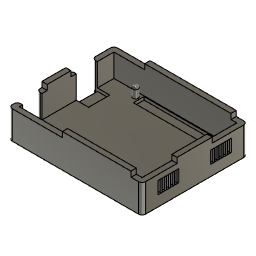
arduino-box-v3 (Autodesk Fusion 360 design; units mm, degrees)
Autodesk Fusion 360 part; units mm, degrees
note: some values were not read from the file. Set by a fixed rule: which sketch regions a step uses.
sketch "Base" plane through (0, 0, 0) normal (0, 0, 1) x (1, 0, 0)
  line L0 (0, 0) -> (75.8, 0)
  line L1 (75.8, 0) -> (75.8, 59.8)
  line L2 (75.8, 59.8) -> (0, 59.8)
  line L3 (0, 59.8) -> (0, 0)
  line L4 (3, 3) -> (72.8, 3)
  line L5 (72.8, 3) -> (72.8, 56.8)
  line L6 (72.8, 56.8) -> (3, 56.8)
  line L7 (3, 56.8) -> (3, 3)
  line L8 (3, 56.8) -> (3, 59.8) construction
  line L9 (3, 56.8) -> (0, 56.8) construction
  line L10 (72.8, 3) -> (72.8, 0) construction
  line L11 (75.8, 3) -> (72.8, 3) construction
  line L12 (3.4, 3.4) -> (72.4, 3.4)
  line L13 (72.4, 3.4) -> (72.4, 56.4)
  line L14 (72.4, 56.4) -> (3.4, 56.4)
  line L15 (3.4, 56.4) -> (3.4, 3.4)
  line L16 (3.4, 56.4) -> (3, 56.4) construction
  line L17 (3.4, 56.4) -> (3.4, 56.8) construction
  line L18 (72.4, 3.4) -> (72.4, 3) construction
  line L19 (72.4, 3.4) -> (72.8, 3.4) construction
  line L20 (3, 13.4) -> (13, 13.4)
  line L21 (13, 13.4) -> (13, 3.4)
  line L22 (0, 15.9) -> (3, 15.9)
  line L23 (0, 4.9) -> (3, 4.9)
  line L24 (0, 47.4) -> (3, 47.4)
  line L25 (0, 35.4) -> (3, 35.4)
  line L26 (3, 47.4) -> (10, 47.4)
  line L27 (10, 47.4) -> (10, 35.4)
  line L28 (10, 35.4) -> (3, 35.4)
  line L29 (20.5, 56.4) -> (20.5, 50.4)
  line L30 (20.5, 50.4) -> (69.5, 50.4)
  line L31 (69.5, 50.4) -> (69.5, 56.4)
  line L32 (30.5, 3.4) -> (30.5, 9.4)
  line L33 (30.5, 9.4) -> (69.5, 9.4)
  line L34 (69.5, 9.4) -> (69.5, 3.4)
  line L35 (72.4, 35.4) -> (66.4, 35.4)
  line L36 (66.4, 35.4) -> (66.4, 26.4)
  line L37 (66.4, 26.4) -> (72.4, 26.4)
  circle A0 centre (18.2, 53.86) radius 1.5
  circle A1 centre (70, 38.4) radius 1.5
  circle A2 centre (70, 10.4) radius 1.5
  line L38 (3.4, 3.4) -> (3, 3.4)
  dimension "d9" = 3
  dimension "d10" = 0.4
  dimension "d11" = 53
  dimension "d12" = 69
  dimension "charging_hole_length" = 10
  dimension "charging_space" = 11
  dimension "charging_y_coord" = 4.9
  dimension "usb_space" = 12
  dimension "usb_y_coord" = 35.4
  dimension "usb_hole_length" = 7
  dimension "d19" = 6
  dimension "pin_row_1_length" = 49
  dimension "pin_row_1_x_coord" = 20.5
  dimension "d22" = 6
  dimension "pin_row_2_length" = 39
  dimension "pin_row_2_x_coord" = 30.5
  dimension "centered_pins_length" = 9
  dimension "d26" = 6
  dimension "centered_pins_y_coord" = 26.4
  dimension "d28" = 3
  dimension "circle_1_x_coord" = 18.2
  dimension "circle_1_space_to_top" = 2.54
  dimension "circle_2_y_coord" = 38.4
  dimension "circle_3_y_coord" = 10.4
  dimension "circle_2_x_coord" = 70
  dimension "circle_3_x_coord" = 70
  constraint horizontal L0
  constraint vertical L1
  constraint horizontal L2
  constraint vertical L3
  constraint coincident L0.start L3.end
  constraint horizontal L4
  constraint vertical L5
  constraint horizontal L6
  constraint vertical L7
  constraint coincident L2 L8.end
  constraint perpendicular L6 L8
  constraint coincident L3 L9.end
  constraint perpendicular L3 L9
  constraint coincident L0 L10.end
  constraint perpendicular L0 L10
  constraint coincident L1 L11.start
  constraint perpendicular L5 L11
  constraint equal L8 L9
  constraint equal L8 L11
  constraint equal L8 L10
  constraint horizontal L12
  constraint vertical L13
  constraint horizontal L14
  constraint vertical L15
  constraint coincident L7 L16.end
  constraint perpendicular L7 L16
  constraint coincident L6 L17.end
  constraint perpendicular L6 L17
  constraint coincident L4 L18.end
  constraint perpendicular L4 L18
  constraint coincident L5 L19.end
  constraint perpendicular L5 L19
  constraint equal L16 L17
  constraint equal L17 L19
  constraint equal L17 L18
  constraint coincident L7 L20.start
  constraint perpendicular L15 L20
  constraint coincident L12 L21.end
  constraint perpendicular L12 L21
  constraint equal L20 L21
  constraint coincident L3 L22.start
  constraint coincident L7 L22.end
  constraint perpendicular L7 L22
  constraint coincident L3 L23.start
  constraint coincident L7 L23.end
  constraint perpendicular L7 L23
  constraint coincident L3 L24.start
  constraint coincident L7 L24.end
  constraint perpendicular L7 L24
  constraint coincident L3 L25.start
  constraint coincident L7 L25.end
  constraint perpendicular L7 L25
  constraint perpendicular L15 L26
  constraint perpendicular L26 L27
  constraint perpendicular L27 L28
  constraint coincident L14 L29.start
  constraint perpendicular L14 L29
  constraint perpendicular L29 L30
  constraint coincident L14 L31.end
  constraint perpendicular L30 L31
  constraint coincident L12 L32.start
  constraint perpendicular L12 L32
  constraint perpendicular L3 L33
  constraint coincident L12 L34.end
  constraint perpendicular L33 L34
  constraint coincident L13 L35.start
  constraint perpendicular L13 L35
  constraint perpendicular L35 L36
  constraint coincident L13 L37.end
  constraint perpendicular L13 L37
  constraint equal A0 A2
  constraint equal A0 A1
  constraint coincident L7 L38.end
  constraint perpendicular L7 L38
  measures "d9" distance of L6.end L8.end
  measures "d10" distance of L14.end L17.end
  measures "d11" distance of L12.start L14.end
  measures "d12" distance of L13.end L14.end
  measures "charging_hole_length" distance of L20.start L20.end
  measures "charging_space" distance of L22 L23
  measures "charging_y_coord" distance of L0 L23
  measures "usb_space" distance of L24 L25
  measures "usb_y_coord" distance of L0 L25
  measures "usb_hole_length" distance of L24.end L26.end
  measures "d19" distance of L30.end L31.end
  measures "pin_row_1_length" distance of L29.end L30.end
  measures "pin_row_1_x_coord" distance of L3 L29
  measures "d22" distance of L33.end L34.end
  measures "pin_row_2_length" distance of L32.end L33.end
  measures "pin_row_2_x_coord" distance of L3 L32
  measures "centered_pins_length" distance of L35.end L36.end
  measures "d26" distance of L35.start L35.end
  measures "centered_pins_y_coord" distance of L0 L37
  measures "d28" diameter of A0
  measures "circle_1_x_coord" distance of L3 A0.centre
  measures "circle_1_space_to_top" distance of L14 A0.centre
  measures "circle_2_y_coord" distance of L0 A1.centre
  measures "circle_3_y_coord" distance of L0 A2.centre
  measures "circle_2_x_coord" distance of L3 A1.centre
  measures "circle_3_x_coord" distance of L3 A2.centre
extrude "Extrude1" add sketch "Base" along normal blind 3 contours L7 L15 L20 L28 | L4 L5 L6 L7 L12 L13 L14 L15 L26 L38 | L12 L13 L14 L15 L20 L21 L26 L27 L28 L29 L30 L31 L32 L33 L34 L35 L36 L37 A2
extrude "Extrude2" add sketch "Base" along normal blind 16 contours L0 L1 L2 L3 L4 L5 L6 L7 L23 L24 | L3 L7 L22 L25
extrude "Extrude3" add sketch "Base" along normal blind 1.3 contours L7 L15 L20 L38 | L7 L15 L26 L28 | L12 L15 L20 L21 | L15 L26 L27 L28 | L12 L32 L33 L34 A2 | L14 L29 L30 L31 | L13 L35 L36 L37
extrude "Extrude4" add sketch "Base" along normal blind 9 contours L33 L34 A2 | L33 L34 A2 | A0 | A1
sketch "Ventilation" plane through (75.8, 0, 0) normal (1, 0, 0) x (0, 1, 0)
  line L0 (0, 0) -> (59.8, 0)
  line L1 (59.8, 0) -> (59.8, 16)
  line L2 (59.8, 16) -> (0, 16)
  line L3 (0, 16) -> (0, 0)
  line L4 (0, 3) -> (59.8, 3) construction
  line L5 (0, 0) -> (59.8, 0)
  line L6 (29.9, 16) -> (29.9, 3) construction
  line L7 (29.9, 9.5) -> (0, 9.5) construction
  line L8 (15.55, 13) -> (14.35, 13)
  line L9 (14.35, 13) -> (14.35, 6)
  line L10 (14.35, 6) -> (15.55, 6)
  line L11 (15.55, 6) -> (15.55, 13)
  line L12 (15.55, 13) -> (14.35, 6) construction
  line L13 (14.35, 13) -> (15.55, 6) construction
  line L14 (15.55, 13) -> (16.75, 13) construction
  line L15 (16.75, 13) -> (17.95, 13)
  line L16 (17.95, 13) -> (17.95, 6)
  line L17 (17.95, 6) -> (16.75, 6)
  line L18 (16.75, 6) -> (16.75, 13)
  line L19 (17.95, 13) -> (19.15, 13) construction
  line L20 (19.15, 13) -> (20.35, 13)
  line L21 (20.35, 13) -> (20.35, 6)
  line L22 (20.35, 6) -> (19.15, 6)
  line L23 (19.15, 6) -> (19.15, 13)
  line L24 (14.35, 13) -> (13.15, 13) construction
  line L25 (13.15, 13) -> (11.95, 13)
  line L26 (11.95, 13) -> (11.95, 6)
  line L27 (11.95, 6) -> (13.15, 6)
  line L28 (13.15, 6) -> (13.15, 13)
  line L29 (11.95, 13) -> (10.75, 13) construction
  line L30 (10.75, 13) -> (9.55, 13)
  line L31 (9.55, 13) -> (9.55, 6)
  line L32 (9.55, 6) -> (10.75, 6)
  line L33 (10.75, 6) -> (10.75, 13)
  line L34 (40.65, 13) -> (39.45, 13)
  line L35 (40.65, 6) -> (40.65, 13)
  line L36 (39.45, 13) -> (39.45, 6)
  line L37 (39.45, 6) -> (40.65, 6)
  line L38 (41.85, 13) -> (41.85, 6)
  line L39 (41.85, 6) -> (43.05, 6)
  line L40 (43.05, 6) -> (43.05, 13)
  line L41 (43.05, 13) -> (41.85, 13)
  line L42 (44.25, 6) -> (44.25, 13)
  line L43 (45.45, 13) -> (45.45, 6)
  line L44 (45.45, 6) -> (44.25, 6)
  line L45 (44.25, 13) -> (45.45, 13)
  line L46 (46.65, 6) -> (46.65, 13)
  line L47 (47.85, 13) -> (47.85, 6)
  line L48 (46.65, 13) -> (47.85, 13)
  line L49 (49.05, 13) -> (50.25, 13)
  line L50 (49.05, 6) -> (49.05, 13)
  line L51 (50.25, 13) -> (50.25, 6)
  line L52 (50.25, 6) -> (49.05, 6)
  line L53 (47.85, 6) -> (46.65, 6)
  point P0 (14.95, 9.5)
  dimension "d43" = 3
  dimension "ventilation_height" = 7
  dimension "ventilation_width" = 1.2
  constraint coincident L3 L4.start
  constraint coincident L1 L4.end
  constraint perpendicular L1 L4
  constraint midpoint L2 L6.start
  constraint midpoint L4 L6.end
  constraint midpoint L6 L7.start
  constraint coincident L3 L7.end
  constraint perpendicular L6 L7
  constraint horizontal L8
  constraint perpendicular L8 L9
  constraint parallel L8 L10
  constraint parallel L9 L11
  constraint coincident L12 P0
  constraint coincident L13 P0
  constraint midpoint L7 P0
  constraint perpendicular L11 L14
  constraint horizontal L15
  constraint vertical L16
  constraint horizontal L17
  constraint vertical L18
  constraint perpendicular L16 L19
  constraint horizontal L20
  constraint vertical L21
  constraint horizontal L22
  constraint vertical L23
  constraint perpendicular L9 L24
  constraint horizontal L25
  constraint vertical L26
  constraint horizontal L27
  constraint vertical L28
  constraint perpendicular L26 L29
  constraint horizontal L30
  constraint vertical L31
  constraint horizontal L32
  constraint vertical L33
  constraint equal L8 L30
  constraint equal L8 L29
  constraint equal L8 L25
  constraint equal L8 L24
  constraint coincident L14.end L15.start
  constraint equal L8 L14
  constraint equal L8 L15
  constraint equal L8 L19
  constraint equal L8 L20
  constraint equal L9 L28
  constraint equal L9 L33
  constraint equal L11 L18
  constraint equal L11 L23
  constraint symmetric L6 L8.start L42.end
  constraint symmetric L6 L8.end L43.start
  constraint symmetric L6 L9.end L43.end
  constraint symmetric L6 L10.end L42.start
  constraint symmetric L6 L14.end L40.end
  constraint symmetric L6 L15.end L38.start
  constraint symmetric L6 L16.end L38.end
  constraint symmetric L6 L17.end L39.end
  constraint symmetric L6 L19.end L34.start
  constraint symmetric L6 L20.end L34.end
  constraint symmetric L6 L21.end L36.end
  constraint symmetric L6 L22.end L35.start
  constraint symmetric L6 L24.end L46.end
  constraint symmetric L6 L25.end L47.start
  constraint symmetric L6 L26.end L47.end
  constraint symmetric L6 L27.end L46.start
  constraint symmetric L6 L29.end L49.start
  constraint symmetric L6 L30.end L49.end
  constraint symmetric L6 L31.end L51.end
  constraint symmetric L6 L32.end L50.start
  measures "d43" distance of L4 L5
  measures "ventilation_height" distance of L8.end L9.end
  measures "ventilation_width" distance of L8.start L8.end
extrude "Extrude5" cut sketch "Ventilation" against normal blind 3 contours L8 L9 L10 L11 | L15 L16 L17 L18 | L20 L21 L22 L23 | L25 L26 L27 L28 | L30 L31 L32 L33 | L34 L35 L36 L37 | L38 L39 L40 L41 | L42 L43 L44 L45 | L46 L47 L48 L53 | L49 L50 L51 L52
fillet "Fillet1" radius 0.5 40 edges at (75.8, 20.35, 9.5) (75.8, 19.15, 9.5) (75.8, 17.95, 9.5) (72.8, 20.35, 9.5) (75.8, 16.75, 9.5) (72.8, 19.15, 9.5) (75.8, 15.55, 9.5) (72.8, 17.95, 9.5) (72.8, 16.75, 9.5) (75.8, 14.35, 9.5) (75.8, 13.15, 9.5) (72.8, 15.55, 9.5) (75.8, 11.95, 9.5) (72.8, 14.35, 9.5) (75.8, 10.75, 9.5) (72.8, 13.15, 9.5) (75.8, 9.55, 9.5) (72.8, 11.95, 9.5) (72.8, 10.75, 9.5) (72.8, 9.55, 9.5) (75.8, 50.25, 9.5) (75.8, 49.05, 9.5) (72.8, 50.25, 9.5) (75.8, 47.85, 9.5) (72.8, 49.05, 9.5) (75.8, 46.65, 9.5) (72.8, 47.85, 9.5) (75.8, 45.45, 9.5) (72.8, 46.65, 9.5) (75.8, 44.25, 9.5) (72.8, 45.45, 9.5) (75.8, 43.05, 9.5) (72.8, 44.25, 9.5) (75.8, 41.85, 9.5) (72.8, 43.05, 9.5) (75.8, 40.65, 9.5) (72.8, 41.85, 9.5) (75.8, 39.45, 9.5) (72.8, 40.65, 9.5) (72.8, 39.45, 9.5)
sketch "Teeth" plane through (0, 0, 16) normal (0, 0, 1) x (-1, 0, 0)
  line L0 (0, -4.9) -> (0, 0)
  line L1 (0, 0) -> (-75.8, 0)
  line L2 (-75.8, 0) -> (-75.8, -59.8)
  line L3 (-75.8, -59.8) -> (0, -59.8)
  line L4 (0, -59.8) -> (0, -47.4)
  line L5 (0, -47.4) -> (-3, -47.4)
  line L6 (-3, -47.4) -> (-3, -56.8)
  line L7 (-3, -56.8) -> (-72.8, -56.8)
  line L8 (-72.8, -56.8) -> (-72.8, -3)
  line L9 (-72.8, -3) -> (-3, -3)
  line L10 (-3, -3) -> (-3, -4.9)
  line L11 (-3, -4.9) -> (0, -4.9)
  line L12 (-20.5, -59.8) -> (-20.5, -56.8)
  line L13 (-69.5, -59.8) -> (-69.5, -56.8)
  line L14 (0, -59.8) -> (0, 0)
  line L15 (-20.5, -59.8) -> (-69.5, -59.8)
  line L16 (-20.5, -56.8) -> (-69.5, -56.8)
  line L17 (-72.8, -39.9) -> (-75.8, -39.9)
  line L18 (-75.8, -39.9) -> (-75.8, -19.9)
  line L19 (-75.8, -19.9) -> (-72.8, -19.9)
  line L20 (-72.8, -19.9) -> (-72.8, -39.9)
  line L21 (-75.8, 0) -> (-75.8, -59.8)
  line L22 (0, -32.4) -> (-3, -32.4)
  line L23 (-3, -32.4) -> (-3, -18.9)
  line L24 (-3, -18.9) -> (0, -18.9)
  line L25 (0, -32.4) -> (0, -18.9)
  line L26 (-30.5, 0) -> (-30.5, -3)
  line L27 (-30.5, -3) -> (-69.5, -3)
  line L28 (-69.5, -3) -> (-69.5, 0)
  line L29 (-69.5, 0) -> (-30.5, 0)
  point P0 (0, -35.4)
  point P1 (0, -15.9)
  dimension "d52" = 49
  dimension "d53" = 20.5
  dimension "back_tooth_length" = 20
  dimension "d55" = 3
  dimension "front_tooth_padding" = 3
  dimension "d57" = 3
  dimension "d58" = 39
  dimension "d59" = 30.5
  constraint coincident L3 L12.start
  constraint coincident L7 L12.end
  constraint perpendicular L7 L12
  constraint coincident L3 L13.start
  constraint coincident L7 L13.end
  constraint perpendicular L7 L13
  constraint horizontal L17
  constraint vertical L18
  constraint horizontal L19
  constraint vertical L20
  constraint coincident L2 L18.end
  constraint coincident L8 L17.start
  constraint midpoint L18 L21
  constraint coincident L14 L22.start
  constraint perpendicular L14 L22
  constraint coincident L14 L24.end
  constraint perpendicular L14 L24
  constraint perpendicular L23 L24
  constraint coincident L1 L26.start
  constraint coincident L9 L26.end
  constraint perpendicular L9 L26
  constraint coincident L9 L27.end
  constraint perpendicular L26 L27
  constraint coincident L1 L28.end
  constraint perpendicular L1 L28
  measures "d52" distance of L12 L13
  measures "d53" distance of L12 L14
  measures "back_tooth_length" distance of L17 L19
  measures "d55" distance of L22.start L22.end
  measures "front_tooth_padding" distance of L22 P0
  measures "d57" distance of L24 P1
  measures "d58" distance of L26 L28
  measures "d59" distance of L14 L26
extrude "Extrude6" add sketch "Teeth" along normal blind 3 contours L14 L22 L23 L24 L25 | L1 L9 L26 L27 L28 L29 | L2 L8 L17 L18 L19 L20 L21 | L3 L7 L12 L13 L15 L16
sketch "Plexi" plane through (0, 0, 16) normal (0, 0, 1) x (-1, 0, 0)
  line L0 (-20.5, -56.8) -> (-20.5, -59.8)
  line L1 (-20.5, -59.8) -> (0, -59.8)
  line L2 (0, -59.8) -> (0, -47.4)
  line L3 (0, -47.4) -> (-3, -47.4)
  line L4 (-3, -47.4) -> (-3, -56.8)
  line L5 (-3, -56.8) -> (-20.5, -56.8)
  line L6 (0, -32.4) -> (0, -59.8)
  line L7 (0, -59.8) -> (-20.5, -59.8)
  line L8 (-20.5, -59.8) -> (-20.5, -50.4)
  line L9 (-20.5, -50.4) -> (-69.5, -50.4)
  line L10 (-69.5, -50.4) -> (-69.5, -59.8)
  line L11 (-69.5, -59.8) -> (-75.8, -59.8)
  line L12 (-75.8, -59.8) -> (-75.8, -39.9)
  line L13 (-75.8, -39.9) -> (-72.8, -39.9)
  line L14 (-72.8, -39.9) -> (-72.8, -35.4)
  line L15 (-72.8, -35.4) -> (-66.4, -35.4)
  line L16 (-66.4, -35.4) -> (-66.4, -26.4)
  line L17 (-66.4, -26.4) -> (-72.8, -26.4)
  line L18 (-72.8, -26.4) -> (-72.8, -19.9)
  line L19 (-72.8, -19.9) -> (-75.8, -19.9)
  line L20 (-75.8, -19.9) -> (-75.8, 0)
  line L21 (-75.8, 0) -> (-69.5, 0)
  line L22 (-69.5, 0) -> (-69.5, -9.4)
  line L23 (-69.5, -9.4) -> (-30.5, -9.4)
  line L24 (-30.5, -9.4) -> (-30.5, 0)
  line L25 (-30.5, 0) -> (0, 0)
  line L26 (0, 0) -> (0, -18.9)
  line L27 (0, -18.9) -> (-3, -18.9)
  line L28 (-3, -18.9) -> (-3, -32.4)
  line L29 (-3, -32.4) -> (0, -32.4)
  point P0 (-75.8, -59.8)
  point P1 (-69.5, -59.8)
  point P2 (-69.5, -50.4)
  point P3 (-3, -32.4)
  point P4 (-3, -18.9)
  point P5 (-30.5, -9.4)
  point P6 (-69.5, 0)
  point P7 (-75.8, 0)
  point P8 (-72.8, -19.9)
  point P9 (-66.4, -26.4)
  point P10 (-72.8, -39.9)
  point P11 (-66.4, -35.4)
  constraint coincident L1.end L2.start
  constraint coincident L0.end L1.start
  constraint perpendicular L7 L8
  constraint perpendicular L8 L9
  constraint perpendicular L9 L10
  constraint perpendicular L10 L11
  constraint perpendicular L11 L12
  constraint perpendicular L10 L13
  constraint perpendicular L13 L14
  constraint perpendicular L14 L15
  constraint perpendicular L15 L16
  constraint perpendicular L16 L17
  constraint perpendicular L17 L18
  constraint perpendicular L18 L19
  constraint perpendicular L19 L20
  constraint perpendicular L20 L21
  constraint perpendicular L19 L22
  constraint perpendicular L20 L23
  constraint perpendicular L23 L24
  constraint coincident L25.end L26.start
  constraint perpendicular L24 L25
  constraint perpendicular L25 L26
  constraint perpendicular L26 L27
  constraint perpendicular L27 L28
  constraint perpendicular L28 L29
  constraint vertical L6
  constraint coincident L6.start L29.end
  constraint coincident P0 L11.end
  constraint coincident P1 L10.end
  constraint coincident P2 L9.end
  constraint coincident P3 L28.end
  constraint coincident P4 L27.end
  constraint coincident P5 L23.end
  constraint coincident P6 L21.end
  constraint coincident P7 L20.end
  constraint coincident P8 L18.end
  constraint coincident P9 L16.end
  constraint coincident P10 L13.end
  constraint coincident P11 L15.end
fillet "Fillet2" radius 2 8 edges at (0, 0, 8) (0, 4.9, 8) (0, 15.9, 8) (0, 35.4, 8) (0, 47.4, 8) (0, 59.8, 8) (75.8, 59.8, 8) (75.8, 0, 8)
fillet "Fillet3" radius 1.5 3 edges at (68.6015, 37.8576, 9) (68.6015, 9.8576, 9) (16.8015, 53.3176, 9)
equation "arduino_length = 69 mm"
equation "arduino_width = 53 mm"
equation "tolerance = 0.4 mm"
equation "thikness = 3 mm"
equation "circle_diam = 3.2 mm - circle_tolerance"
equation "circle_tolerance = 0.2 mm"
equation "pin_row_width = 6 mm"
equation "d9 = thikness"
equation "d10 = tolerance"
equation "d11 = arduino_width"
equation "d12 = arduino_length"
equation "charging_y_coord = thikness + tolerance + 1.5 mm"
equation "usb_y_coord = thikness + tolerance + 32 mm"
equation "d19 = pin_row_width"
equation "pin_row_1_x_coord = thikness + tolerance + 17.1 mm"
equation "d22 = pin_row_width"
equation "pin_row_2_x_coord = thikness + tolerance + 27.1 mm"
equation "d26 = pin_row_width"
equation "centered_pins_y_coord = thikness + tolerance + 23 mm"
equation "d28 = circle_diam"
equation "circle_1_x_coord = thikness + circle_tolerance + 15 mm"
equation "circle_2_y_coord = thikness + tolerance + 35 mm"
equation "circle_3_y_coord = thikness + tolerance + 7 mm"
equation "circle_2_x_coord = thikness + tolerance + 66.6 mm"
equation "circle_3_x_coord = circle_2_x_coord"
equation "d35 = thikness"
equation "d37 = thikness + 13 mm"
equation "hole_thikness = 1.3 mm"
equation "circle_height = 3 * thikness"
equation "d43 = thikness"
equation "d46 = -thikness"
equation "d52 = pin_row_1_length"
equation "d53 = pin_row_1_x_coord"
equation "d55 = thikness"
equation "d57 = front_tooth_padding"
equation "d58 = pin_row_2_length"
equation "d59 = pin_row_2_x_coord"
equation "d60 = thikness"
equation "d65 = circle_diam / 2"
